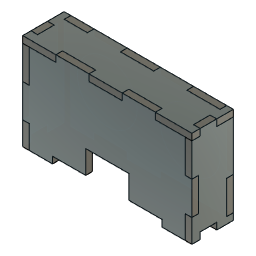
HR-SR04 LASER CUT PART v9 (Autodesk Fusion 360 design; units mm, degrees)
Autodesk Fusion 360 part; units mm, degrees
mesh "Mesh1" [no effect]
ref_plane "WorkPlane1" through (0, -8, 0) normal (0, 1, 0) x (0, 0, 1)
sketch "Sketch2" plane through (0, -8, 0) normal (0, 1, 0) x (1, 0, 0)
  line L0 (23.3967, -21.6051) -> (-23.6033, -21.6051)
  line L1 (-23.6033, -21.6051) -> (-23.6033, 3.3949)
  line L2 (-23.6033, 3.3949) -> (23.3967, 3.3949)
  line L3 (23.3967, 3.3949) -> (23.3967, -21.6051)
  line L4 (-23.6033, -9.1051) -> (-12.6033, -9.1051) construction
  line L5 (-12.6033, -9.1051) -> (-12.6033, 3.3949) construction
  line L6 (23.3967, -9.1051) -> (12.3967, -9.1051) construction
  line L7 (12.3967, -9.1051) -> (12.3967, 3.3949)
  circle A0 centre (12.3967, -9.1051) radius 9
  circle A1 centre (-12.6033, -9.1051) radius 9
  line L8 (23.3967, -21.6051) -> (23.3967, -23.6051)
  line L9 (23.3967, -23.6051) -> (13.3967, -23.6051)
  line L10 (13.3967, -23.6051) -> (13.3967, -21.6051)
  line L11 (13.3967, -21.6051) -> (23.3967, -21.6051)
  line L12 (3.3967, -23.6051) -> (-6.6033, -23.6051)
  line L13 (-6.6033, -23.6051) -> (-6.6033, -21.6051)
  line L14 (-6.6033, -21.6051) -> (3.3967, -21.6051)
  line L15 (3.3967, -21.6051) -> (3.3967, -23.6051)
  line L16 (-6.6033, -23.6051) -> (-16.6033, -23.6051) construction
  line L17 (-16.6033, -23.6051) -> (-16.6033, -21.6051)
  line L18 (-16.6033, -23.6051) -> (-23.6033, -23.6051)
  line L19 (-23.6033, -23.6051) -> (-23.6033, -21.6051)
  line L20 (23.3967, 3.3949) -> (25.3967, 3.3949)
  line L21 (25.3967, 3.3949) -> (25.3967, -6.6051)
  line L22 (25.3967, -6.6051) -> (23.3967, -6.6051)
  line L23 (23.3967, -6.6051) -> (23.3967, 3.3949)
  line L24 (23.3967, 3.3949) -> (23.3967, 5.3949)
  line L25 (23.3967, 5.3949) -> (13.3967, 5.3949)
  line L26 (13.3967, 5.3949) -> (13.3967, 3.3949)
  line L27 (13.3967, 3.3949) -> (23.3967, 3.3949)
  line L28 (3.3967, 5.3949) -> (-6.6033, 5.3949)
  line L29 (-6.6033, 5.3949) -> (-6.6033, 3.3949)
  line L30 (3.3967, 3.3949) -> (3.3967, 5.3949)
  line L31 (-23.6033, 5.3949) -> (-23.6033, 3.3949)
  line L32 (-16.6033, 5.3949) -> (-23.6033, 5.3949)
  line L33 (-16.6033, 5.3949) -> (-16.6033, 3.3949)
  line L34 (-6.6033, 3.3949) -> (3.3967, 3.3949)
  line L35 (-23.6033, -21.6051) -> (-25.6033, -21.6051)
  line L36 (-25.6033, -21.6051) -> (-25.6033, -11.6051)
  line L37 (-25.6033, -11.6051) -> (-23.6033, -11.6051)
  dimension "d2" = 47
  dimension "d3" = 25
  dimension "d4" = 11
  dimension "d5" = 11
  dimension "d6" = 18
  dimension "d7" = 18
  dimension "d14" = 2
  dimension "d15" = 10
  dimension "d16" = 2
  dimension "d20" = -20
  dimension "d21" = 0
  dimension "d25" = 10
  dimension "d26" = 2
  dimension "d30" = 2
  dimension "d31" = 10
  dimension "d37" = 2
  dimension "d38" = 10
  constraint horizontal L0
  constraint vertical L1
  constraint horizontal L2
  constraint vertical L3
  constraint midpoint L1 L4.start
  constraint perpendicular L1 L4
  constraint coincident L2 L5.end
  constraint perpendicular L2 L5
  constraint midpoint L3 L6.start
  constraint perpendicular L3 L6
  constraint coincident L2 L7.end
  constraint perpendicular L2 L7
  constraint coincident L6.end L7.start
  constraint coincident L4.end L5.start
  constraint perpendicular L0 L8
  constraint perpendicular L8 L9
  constraint perpendicular L0 L10
  constraint perpendicular L13 L16
  constraint perpendicular L0 L17
  constraint perpendicular L1 L18
  constraint perpendicular L0 L19
  constraint perpendicular L3 L20
  constraint perpendicular L20 L21
  constraint coincident L3 L22.end
  constraint perpendicular L3 L22
  constraint symmetric L0.start L4 L2.end
  constraint symmetric L0.end L4 L1.end
  constraint symmetric L4 L8.end L24.end
  constraint symmetric L4 L9.end L25.end
  constraint symmetric L4 L10.end L26.end
  constraint symmetric L4 L12.start L28.start
  constraint symmetric L4 L12.end L28.end
  constraint symmetric L4 L13.end L29.end
  constraint symmetric L4 L14.end L30.start
  constraint symmetric L4 L16.end L32.start
  constraint symmetric L4 L17.end L33.end
  constraint symmetric L4 L18.end L31.start
  constraint perpendicular L19 L35
  constraint perpendicular L35 L36
  constraint coincident L1 L37.end
  constraint perpendicular L1 L37
  measures "d2" distance of L0.start L0.end
  measures "d3" distance of L0.end L1.end
  measures "d4" distance of L4.start L4.end
  measures "d5" distance of L6.start L6.end
  measures "d6" diameter of A0
  measures "d7" diameter of A1
  measures "d14" distance of L0.start L8.end
  measures "d15" distance of L8.end L9.end
  measures "d16" distance of L9.end L10.end
  measures "d25" distance of L12.end L16.end
  measures "d26" distance of L16.end L17.end
  measures "d30" distance of L2.end L20.end
  measures "d31" distance of L20.end L21.end
  measures "d37" distance of L0.end L35.end
  measures "d38" distance of L35.end L36.end
extrude "Extrude1" add sketch "Sketch2" along normal blind 2 contours L0 L1 L2 L3 L11 L14 L23 L27 L34 makes body 1
extrude "Extrude2" add sketch "Sketch2" along normal blind 2 contours L0 L8 L9 L10 L11 | L0 L12 L13 L14 L15 bodies 1
extrude "Extrude3" add sketch "Sketch2" along normal blind 2 contours L0 L17 L18 L19 bodies 1
extrude "Extrude4" add sketch "Sketch2" along normal blind 2 contours L3 L20 L21 L22 L23 bodies 1
extrude "Extrude5" add sketch "Sketch2" along normal blind 2 contours L2 L24 L25 L26 L27 | L2 L28 L29 L30 L34 | L2 L31 L32 L33 bodies 1
extrude "Extrude6" add sketch "Sketch2" along normal blind 2 contours L1 L35 L36 L37 bodies 1
sketch "Sketch3" plane through (0, 0, 23.6051) normal (0, 0, 1) x (-1, 0, 0)
  line L0 (6.6033, 8) -> (-3.3967, 8)
  line L1 (-3.3967, 8) -> (-3.3967, 6)
  line L2 (-3.3967, 6) -> (6.6033, 6)
  line L3 (6.6033, 6) -> (6.6033, 8)
  line L4 (25.6033, 6) -> (-25.3967, 6)
  line L5 (-25.3967, 6) -> (-25.3967, 18.5)
  line L6 (-25.3967, 18.5) -> (25.6033, 18.5)
  line L7 (25.6033, 18.5) -> (25.6033, 6)
  line L8 (23.6033, 6) -> (16.6033, 6)
  line L9 (16.6033, 6) -> (16.6033, 8)
  line L10 (16.6033, 8) -> (23.6033, 8)
  line L11 (23.6033, 8) -> (23.6033, 6)
  line L12 (6.6033, 6) -> (-3.3967, 6)
  line L13 (-3.3967, 6) -> (-3.3967, 8)
  line L14 (-3.3967, 8) -> (6.6033, 8)
  line L15 (6.6033, 8) -> (6.6033, 6)
  line L16 (-13.3967, 6) -> (-23.3967, 6)
  line L17 (-23.3967, 6) -> (-23.3967, 8)
  line L18 (-23.3967, 8) -> (-13.3967, 8)
  line L19 (-13.3967, 8) -> (-13.3967, 6)
  line L20 (-25.3967, 6) -> (-25.3967, 11)
  line L21 (-25.3967, 11) -> (-23.3967, 11)
  line L22 (-23.3967, 11) -> (-23.3967, 16)
  line L23 (-23.3967, 16) -> (-25.3967, 16)
  line L24 (25.6033, 6) -> (25.6033, 11)
  line L25 (25.6033, 11) -> (23.6033, 11)
  line L26 (23.6033, 11) -> (23.6033, 16)
  line L27 (23.6033, 16) -> (25.6033, 16)
  line L28 (25.6033, 18.5) -> (15.6033, 18.5)
  line L29 (15.6033, 18.5) -> (15.6033, 16.5)
  line L30 (15.6033, 16.5) -> (5.6033, 16.5)
  line L31 (5.6033, 16.5) -> (5.6033, 18.5)
  line L32 (5.6033, 18.5) -> (-4.3967, 18.5)
  line L33 (-4.3967, 18.5) -> (-4.3967, 16.5)
  line L34 (-4.3967, 16.5) -> (-14.3967, 16.5)
  line L35 (-14.3967, 16.5) -> (-14.3967, 18.5)
  point P0 (25.6033, 6)
  point P1 (-25.3967, 6)
  point P2 (23.6033, 6)
  point P3 (16.6033, 8)
  point P4 (-13.3967, 6)
  point P5 (-23.3967, 8)
  dimension "d42" = 12.5
  dimension "d45" = 5
  dimension "d46" = 2
  dimension "d47" = 5
  dimension "d62" = 5
  dimension "d63" = 2
  dimension "d64" = 5
  dimension "d80" = 10
  dimension "d81" = 2
  dimension "d82" = 10
  dimension "d83" = 10
  dimension "d84" = 2
  dimension "d85" = 10
  constraint horizontal L4
  constraint vertical L5
  constraint horizontal L6
  constraint vertical L7
  constraint coincident P0 L4.start
  constraint coincident P1 L4.end
  constraint horizontal L8
  constraint vertical L9
  constraint horizontal L10
  constraint vertical L11
  constraint coincident P2 L8.start
  constraint coincident P3 L9.end
  constraint horizontal L12
  constraint vertical L13
  constraint horizontal L14
  constraint vertical L15
  constraint coincident L2.end L3.start
  constraint coincident L0.end L1.start
  constraint horizontal L16
  constraint vertical L17
  constraint horizontal L18
  constraint vertical L19
  constraint coincident P4 L16.start
  constraint coincident P5 L17.end
  constraint perpendicular L4 L20
  constraint perpendicular L20 L21
  constraint perpendicular L6 L22
  constraint coincident L5 L23.end
  constraint perpendicular L5 L23
  constraint perpendicular L4 L24
  constraint perpendicular L7 L25
  constraint perpendicular L25 L26
  constraint coincident L7 L27.end
  constraint perpendicular L7 L27
  constraint perpendicular L7 L28
  constraint perpendicular L6 L29
  constraint perpendicular L29 L30
  constraint coincident L6 L31.end
  constraint perpendicular L6 L31
  constraint perpendicular L31 L32
  constraint perpendicular L6 L33
  constraint perpendicular L33 L34
  constraint coincident L6 L35.end
  constraint perpendicular L6 L35
  measures "d42" distance of P1 L5.end
  measures "d45" distance of P1 L20.end
  measures "d46" distance of L20.end L21.end
  measures "d47" distance of L21.end L22.end
  measures "d62" distance of P0 L24.end
  measures "d63" distance of L24.end L25.end
  measures "d64" distance of L25.end L26.end
  measures "d80" distance of L6.end L28.end
  measures "d81" distance of L28.end L29.end
  measures "d82" distance of L29.end L30.end
  measures "d83" distance of L31.end L32.end
  measures "d84" distance of L32.end L33.end
  measures "d85" distance of L33.end L34.end
extrude "Extrude8" add sketch "Sketch3" against normal blind 2 separate body contours L0 L1 L3 L4 L5 L6 L7 L9 L10 L11 L13 L14 L15 L17 L18 L19 L20 L21 L22 L23 L24 L25 L26 L27 L28 L29 L30 L31 L32 L33 L34 L35 | L7 L25 L26 L27 | L6 L29 L30 L31 | L6 L33 L34 L35 makes body 2
sketch "Sketch4" plane through (23.3967, 0, 0) normal (1, 0, 0) x (0, 1, 0)
  line L0 (-8, 6.6051) -> (-6, 6.6051)
  line L1 (-6, 6.6051) -> (-6, 23.6051)
  line L2 (-6, 23.6051) -> (-8, 23.6051)
  line L3 (-8, 23.6051) -> (-8, 6.6051)
  line L4 (-18.5, 23.6051) -> (-6, 23.6051)
  line L5 (-6, 23.6051) -> (-6, -5.3949)
  line L6 (-6, -5.3949) -> (-18.5, -5.3949)
  line L7 (-18.5, -5.3949) -> (-18.5, 23.6051)
  line L8 (-18.5, 23.6051) -> (-16, 23.6051)
  line L9 (-16, 23.6051) -> (-16, 21.6051)
  line L10 (-16, 21.6051) -> (-18.5, 21.6051)
  line L11 (-18.5, 21.6051) -> (-18.5, 23.6051)
  line L12 (-11, 23.6051) -> (-6, 23.6051)
  line L13 (-6, 23.6051) -> (-6, 21.6051)
  line L14 (-6, 21.6051) -> (-11, 21.6051)
  line L15 (-11, 21.6051) -> (-11, 23.6051)
  line L16 (-8, 6.6051) -> (-6, 6.6051)
  line L17 (-6, 6.6051) -> (-6, -3.3949)
  line L18 (-6, -3.3949) -> (-8, -3.3949)
  line L19 (-8, -3.3949) -> (-8, 6.6051)
  line L20 (-18.5, 21.6051) -> (-18.5, 11.6051)
  line L21 (-18.5, 11.6051) -> (-16.5, 11.6051)
  line L22 (-16.5, 11.6051) -> (-16.5, 1.6051)
  line L23 (-16.5, 1.6051) -> (-18.5, 1.6051)
  line L24 (-6, -5.3949) -> (-11, -5.3949)
  line L25 (-11, -5.3949) -> (-11, -3.3949)
  line L26 (-11, -3.3949) -> (-16, -3.3949)
  line L27 (-16, -3.3949) -> (-16, -5.3949)
  point P0 (-18.5, 23.6051)
  point P1 (-6, 23.6051)
  point P2 (-6, -5.3949)
  point P3 (-16, 21.6051)
  point P4 (-11, 23.6051)
  point P5 (-6, 21.6051)
  point P6 (-6, -3.3949)
  dimension "d52" = 10
  dimension "d53" = 2
  dimension "d54" = 10
  dimension "d55" = 2
  dimension "d58" = 5
  dimension "d59" = 2
  dimension "d77" = 5
  constraint horizontal L4
  constraint vertical L5
  constraint horizontal L6
  constraint vertical L7
  constraint coincident P0 L4.start
  constraint coincident P1 L1.end
  constraint coincident P2 L5.end
  constraint horizontal L8
  constraint vertical L9
  constraint horizontal L10
  constraint vertical L11
  constraint coincident P3 L9.end
  constraint horizontal L12
  constraint vertical L13
  constraint horizontal L14
  constraint vertical L15
  constraint coincident P4 L12.start
  constraint coincident P5 L13.end
  constraint horizontal L16
  constraint vertical L17
  constraint horizontal L18
  constraint vertical L19
  constraint coincident L0.start L3.end
  constraint coincident P6 L17.end
  constraint perpendicular L6 L20
  constraint perpendicular L7 L21
  constraint perpendicular L21 L22
  constraint perpendicular L7 L23
  constraint perpendicular L5 L24
  constraint perpendicular L24 L25
  constraint perpendicular L25 L26
  constraint coincident L6 L27.end
  constraint perpendicular L6 L27
  measures "d52" distance of L10.end L20.end
  measures "d53" distance of L20.end L21.end
  measures "d54" distance of L21.end L22.end
  measures "d55" distance of L22.end L23.end
  measures "d58" distance of P2 L24.end
  measures "d59" distance of L24.end L25.end
  measures "d77" distance of L25.end L26.end
extrude "Extrude12" cut sketch "Sketch3" against normal blind 2 contours L7 L25 L26 L27 bodies 2
ref_plane "WorkPlane2" through (-0.1033, -17.25, 22.6051) normal (1, 0, 0) x (0, -1, 0)
sketch "Sketch5" plane through (-23.6033, 0, 0) normal (-1, 0, 0) x (0, -1, 0)
  line L0 (16, 23.6051) -> (11, 23.6051)
  line L1 (11, 23.6051) -> (11, 21.6051)
  line L2 (11, 21.6051) -> (16, 21.6051)
  line L3 (16, 21.6051) -> (16, 23.6051)
  line L4 (6, 23.6051) -> (18.5, 23.6051)
  line L5 (18.5, 23.6051) -> (18.5, -5.3949)
  line L6 (18.5, -5.3949) -> (6, -5.3949)
  line L7 (6, -5.3949) -> (6, 23.6051)
  line L8 (6, 11.6051) -> (8, 11.6051)
  line L9 (8, 11.6051) -> (8, 21.6051)
  line L10 (8, 21.6051) -> (6, 21.6051)
  line L11 (6, 21.6051) -> (6, 11.6051)
  line L12 (11, 21.6051) -> (6, 21.6051)
  line L13 (6, 21.6051) -> (6, 23.6051)
  line L14 (6, 23.6051) -> (11, 23.6051)
  line L15 (11, 23.6051) -> (11, 21.6051)
  line L16 (16, 21.6051) -> (18.5, 21.6051)
  line L17 (18.5, 21.6051) -> (18.5, 23.6051)
  line L18 (18.5, 23.6051) -> (16, 23.6051)
  line L19 (16, 23.6051) -> (16, 21.6051)
  line L20 (6, -5.3949) -> (11, -5.3949)
  line L21 (11, -5.3949) -> (11, -3.3949)
  line L22 (11, -3.3949) -> (16, -3.3949)
  line L23 (16, -3.3949) -> (16, -5.3949)
  line L24 (18.5, 21.6051) -> (18.5, 11.6051)
  line L25 (18.5, 11.6051) -> (16.5, 11.6051)
  line L26 (16.5, 11.6051) -> (16.5, 1.6051)
  line L27 (16.5, 1.6051) -> (18.5, 1.6051)
  point P0 (6, -5.3949)
  point P1 (18.5, 23.6051)
  point P2 (8, 11.6051)
  dimension "d69" = 5
  dimension "d70" = 2
  dimension "d71" = 5
  dimension "d72" = 10
  dimension "d73" = 2
  dimension "d74" = 10
  constraint horizontal L4
  constraint vertical L5
  constraint horizontal L6
  constraint vertical L7
  constraint coincident P0 L6.end
  constraint coincident P1 L4.end
  constraint horizontal L8
  constraint vertical L9
  constraint horizontal L10
  constraint vertical L11
  constraint coincident L7 L8.start
  constraint horizontal L12
  constraint vertical L13
  constraint horizontal L14
  constraint vertical L15
  constraint coincident L1.end L2.start
  constraint horizontal L16
  constraint vertical L17
  constraint horizontal L18
  constraint vertical L19
  constraint coincident L2.end L3.start
  constraint coincident L4.start L7.end
  constraint coincident P2 L8.end
  constraint coincident L9.end L12
  constraint perpendicular L7 L20
  constraint perpendicular L6 L21
  constraint perpendicular L21 L22
  constraint coincident L6 L23.end
  constraint perpendicular L6 L23
  constraint perpendicular L16 L24
  constraint perpendicular L24 L25
  constraint perpendicular L25 L26
  constraint coincident L5 L27.end
  constraint perpendicular L5 L27
  measures "d69" distance of P0 L20.end
  measures "d70" distance of L20.end L21.end
  measures "d71" distance of L21.end L22.end
  measures "d72" distance of L16.end L24.end
  measures "d73" distance of L24.end L25.end
  measures "d74" distance of L25.end L26.end
extrude "Extrude13" add sketch "Sketch5" along normal blind 2 separate body contours L0 L1 L2 L3 L4 L15 L19 | L2 L5 L6 L7 L8 L9 L12 L16 L20 L21 L22 L23 L24 L25 L26 L27 makes body 3
extrude "Extrude14" add sketch "Sketch4" along normal blind 2 separate body contours L0 L1 L3 L5 L14 L16 | L3 L4 L5 L6 L7 L9 L10 L14 L15 L18 L19 L20 L21 L22 L23 L24 L25 L26 L27 makes body 4
extrude "Extrude15" cut sketch "Sketch3" against normal blind 2 contours L6 L29 L30 L31 | L6 L33 L34 L35 bodies 2
sketch "Sketch7" plane through (0, -16.5, 0) normal (0, -1, 0) x (1, 0, 0)
  line L0 (-23.6033, 1.6051) -> (-23.6033, 11.6051)
  line L1 (-23.6033, 11.6051) -> (-25.6033, 11.6051)
  line L2 (-25.6033, 11.6051) -> (-25.6033, 1.6051)
  line L3 (-25.6033, 1.6051) -> (-23.6033, 1.6051)
  line L4 (-25.6033, 23.6051) -> (25.3967, 23.6051)
  line L5 (25.3967, 23.6051) -> (25.3967, -5.3949)
  line L6 (-25.6033, -5.3949) -> (-25.6033, 23.6051)
  line L7 (-25.6033, 11.6051) -> (-23.6033, 11.6051)
  line L8 (-23.6033, 11.6051) -> (-23.6033, 21.6051)
  line L9 (-23.6033, 21.6051) -> (-25.6033, 21.6051)
  line L10 (-25.6033, 21.6051) -> (-25.6033, 11.6051)
  line L11 (-25.6033, 21.6051) -> (-15.6033, 21.6051)
  line L12 (-15.6033, 21.6051) -> (-15.6033, 23.6051)
  line L13 (-15.6033, 23.6051) -> (-25.6033, 23.6051)
  line L14 (-25.6033, 23.6051) -> (-25.6033, 21.6051)
  line L15 (-5.6033, 23.6051) -> (4.3967, 23.6051)
  line L16 (4.3967, 23.6051) -> (4.3967, 21.6051)
  line L17 (4.3967, 21.6051) -> (-5.6033, 21.6051)
  line L18 (-5.6033, 21.6051) -> (-5.6033, 23.6051)
  line L19 (14.3967, 23.6051) -> (25.3967, 23.6051)
  line L20 (25.3967, 23.6051) -> (25.3967, 21.6051)
  line L21 (25.3967, 21.6051) -> (14.3967, 21.6051)
  line L22 (14.3967, 21.6051) -> (14.3967, 23.6051)
  line L23 (23.3967, 21.6051) -> (25.3967, 21.6051)
  line L24 (25.3967, 21.6051) -> (25.3967, 11.6051)
  line L25 (25.3967, 11.6051) -> (23.3967, 11.6051)
  line L26 (23.3967, 11.6051) -> (23.3967, 21.6051)
  line L27 (23.3967, 1.6051) -> (25.3967, 1.6051)
  line L28 (25.3967, 1.6051) -> (25.3967, -5.3949)
  line L29 (25.3967, -5.3949) -> (23.3967, -5.3949)
  line L30 (23.3967, -5.3949) -> (23.3967, 1.6051)
  line L31 (-25.6033, -5.3949) -> (-23.6033, -5.3949)
  line L32 (-23.6033, -5.3949) -> (-23.6033, 1.6051)
  line L33 (-23.6033, 1.6051) -> (-25.6033, 1.6051)
  line L34 (-25.6033, 1.6051) -> (-25.6033, -5.3949)
  line L35 (6.3967, 3.6051) -> (-6.6033, 3.6051)
  line L36 (-6.6033, 3.6051) -> (-6.6033, -5.3949)
  line L37 (-0.1033, 23.6051) -> (-0.1033, 3.6051) construction
  line L38 (6.3967, 3.6051) -> (6.3967, -5.3949)
  line L39 (-25.6033, -5.3949) -> (25.3967, -5.3949)
  line L40 (-6.6033, -5.3949) -> (-16.6033, -5.3949)
  line L41 (-16.6033, -5.3949) -> (-16.6033, -3.3949)
  line L42 (-16.6033, -3.3949) -> (-6.6033, -3.3949)
  line L43 (-6.6033, -3.3949) -> (-6.6033, -5.3949)
  line L44 (6.3967, -5.3949) -> (16.3967, -5.3949)
  line L45 (16.3967, -5.3949) -> (16.3967, -3.3949)
  line L46 (16.3967, -3.3949) -> (6.3967, -3.3949)
  line L47 (6.3967, -3.3949) -> (6.3967, -5.3949)
  point P0 (-25.6033, 23.6051)
  point P1 (25.3967, -5.3949)
  point P2 (-23.6033, 21.6051)
  point P3 (-15.6033, 23.6051)
  point P4 (-5.6033, 21.6051)
  point P5 (4.3967, 23.6051)
  point P6 (14.3967, 21.6051)
  point P7 (23.3967, 21.6051)
  point P8 (25.3967, 11.6051)
  point P9 (23.3967, 1.6051)
  dimension "d96" = 20
  dimension "d97" = 13
  dimension "d98" = 10
  dimension "d99" = 2
  dimension "d100" = 10
  dimension "d101" = 2
  constraint horizontal L4
  constraint vertical L5
  constraint vertical L6
  constraint coincident P0 L4.start
  constraint coincident P1 L5.end
  constraint horizontal L7
  constraint vertical L8
  constraint horizontal L9
  constraint vertical L10
  constraint coincident L1.end L2.start
  constraint coincident P2 L8.end
  constraint horizontal L11
  constraint vertical L12
  constraint horizontal L13
  constraint vertical L14
  constraint coincident P3 L12.end
  constraint horizontal L15
  constraint vertical L16
  constraint horizontal L17
  constraint vertical L18
  constraint coincident P4 L17.end
  constraint coincident P5 L15.end
  constraint horizontal L19
  constraint vertical L20
  constraint horizontal L21
  constraint vertical L22
  constraint coincident P6 L21.end
  constraint coincident L4.end L5.start
  constraint horizontal L23
  constraint vertical L24
  constraint horizontal L25
  constraint vertical L26
  constraint coincident P7 L23.start
  constraint coincident P8 L24.end
  constraint horizontal L27
  constraint vertical L28
  constraint horizontal L29
  constraint vertical L30
  constraint coincident P9 L27.start
  constraint horizontal L31
  constraint vertical L32
  constraint horizontal L33
  constraint vertical L34
  constraint coincident L0.start L3.end
  constraint horizontal L35
  constraint vertical L36
  constraint midpoint L4 L37.start
  constraint midpoint L35 L37.end
  constraint perpendicular L17 L37
  constraint perpendicular L35 L38
  constraint perpendicular L28 L39
  constraint horizontal L40
  constraint vertical L41
  constraint horizontal L42
  constraint vertical L43
  constraint collinear L39 L40
  constraint horizontal L44
  constraint vertical L45
  constraint horizontal L46
  constraint vertical L47
  constraint collinear L39 L44
  measures "d96" distance of L37.start L37.end
  measures "d97" distance of L35.start L35.end
  measures "d98" distance of L36.end L40.end
  measures "d99" distance of L36.end L42.end
  measures "d100" distance of L38.end L44.end
  measures "d101" distance of L38.end L46.end
extrude "Extrude18" add sketch "Sketch7" along normal blind 2 separate body contours L0 L1 L2 L3 L6 L7 L33 | L0 L4 L5 L8 L11 L12 L16 L17 L18 L21 L22 L25 L26 L27 L30 L32 L35 L36 L38 L39 L41 L42 L45 L46 makes body 5
sketch "FRONT_DXF" plane through (0, -6, 0) normal (0, 1, 0) x (-1, 0, 0)
  circle A0 centre (12.6033, 9.1051) radius 9
  circle A1 centre (-12.3967, 9.1051) radius 9
  line L0 (16.6033, 21.6051) -> (6.6033, 21.6051)
  line L1 (6.6033, 21.6051) -> (6.6033, 23.6051)
  line L2 (6.6033, 23.6051) -> (-3.3967, 23.6051)
  line L3 (-3.3967, 23.6051) -> (-3.3967, 21.6051)
  line L4 (-3.3967, 21.6051) -> (-13.3967, 21.6051)
  line L5 (-13.3967, 21.6051) -> (-13.3967, 23.6051)
  line L6 (-13.3967, 23.6051) -> (-23.3967, 23.6051)
  line L7 (-23.3967, 23.6051) -> (-23.3967, 6.6051)
  line L8 (-23.3967, 6.6051) -> (-25.3967, 6.6051)
  line L9 (-25.3967, 6.6051) -> (-25.3967, -3.3949)
  line L10 (-25.3967, -3.3949) -> (-23.3967, -3.3949)
  line L11 (-23.3967, -3.3949) -> (-23.3967, -5.3949)
  line L12 (-23.3967, -5.3949) -> (-13.3967, -5.3949)
  line L13 (-13.3967, -5.3949) -> (-13.3967, -3.3949)
  line L14 (-13.3967, -3.3949) -> (-3.3967, -3.3949)
  line L15 (-3.3967, -3.3949) -> (-3.3967, -5.3949)
  line L16 (-3.3967, -5.3949) -> (6.6033, -5.3949)
  line L17 (6.6033, -5.3949) -> (6.6033, -3.3949)
  line L18 (6.6033, -3.3949) -> (16.6033, -3.3949)
  line L19 (16.6033, -3.3949) -> (16.6033, -5.3949)
  line L20 (16.6033, -5.3949) -> (23.6033, -5.3949)
  line L21 (23.6033, -5.3949) -> (23.6033, 11.6051)
  line L22 (23.6033, 11.6051) -> (25.6033, 11.6051)
  line L23 (25.6033, 11.6051) -> (25.6033, 21.6051)
  line L24 (25.6033, 21.6051) -> (23.6033, 21.6051)
  line L25 (23.6033, 21.6051) -> (23.6033, 23.6051)
  line L26 (23.6033, 23.6051) -> (16.6033, 23.6051)
  line L27 (16.6033, 23.6051) -> (16.6033, 21.6051)
sketch "LEFT_DXF" plane through (25.3967, 0, 0) normal (1, 0, 0) x (0, 1, 0)
  line L0 (-6, -3.3949) -> (-8, -3.3949)
  line L1 (-8, -3.3949) -> (-8, 6.6051)
  line L2 (-8, 6.6051) -> (-6, 6.6051)
  line L3 (-6, 6.6051) -> (-6, 21.6051)
  line L4 (-6, 21.6051) -> (-11, 21.6051)
  line L5 (-11, 21.6051) -> (-11, 23.6051)
  line L6 (-11, 23.6051) -> (-16, 23.6051)
  line L7 (-16, 23.6051) -> (-16, 21.6051)
  line L8 (-16, 21.6051) -> (-18.5, 21.6051)
  line L9 (-18.5, 21.6051) -> (-18.5, 11.6051)
  line L10 (-18.5, 11.6051) -> (-16.5, 11.6051)
  line L11 (-16.5, 11.6051) -> (-16.5, 1.6051)
  line L12 (-16.5, 1.6051) -> (-18.5, 1.6051)
  line L13 (-18.5, 1.6051) -> (-18.5, -5.3949)
  line L14 (-18.5, -5.3949) -> (-16, -5.3949)
  line L15 (-16, -5.3949) -> (-16, -3.3949)
  line L16 (-16, -3.3949) -> (-11, -3.3949)
  line L17 (-11, -3.3949) -> (-11, -5.3949)
  line L18 (-11, -5.3949) -> (-6, -5.3949)
  line L19 (-6, -5.3949) -> (-6, -3.3949)
sketch "RIGHT_DXF" plane through (-25.6033, 0, 0) normal (-1, 0, 0) x (0, -1, 0)
  line L0 (11, 23.6051) -> (11, 21.6051)
  line L1 (11, 21.6051) -> (8, 21.6051)
  line L2 (8, 21.6051) -> (8, 11.6051)
  line L3 (8, 11.6051) -> (6, 11.6051)
  line L4 (6, 11.6051) -> (6, -5.3949)
  line L5 (6, -5.3949) -> (11, -5.3949)
  line L6 (11, -5.3949) -> (11, -3.3949)
  line L7 (11, -3.3949) -> (16, -3.3949)
  line L8 (16, -3.3949) -> (16, -5.3949)
  line L9 (16, -5.3949) -> (18.5, -5.3949)
  line L10 (18.5, -5.3949) -> (18.5, 1.6051)
  line L11 (18.5, 1.6051) -> (16.5, 1.6051)
  line L12 (16.5, 1.6051) -> (16.5, 11.6051)
  line L13 (16.5, 11.6051) -> (18.5, 11.6051)
  line L14 (18.5, 11.6051) -> (18.5, 21.6051)
  line L15 (18.5, 21.6051) -> (16, 21.6051)
  line L16 (16, 21.6051) -> (16, 23.6051)
  line L17 (16, 23.6051) -> (11, 23.6051)
sketch "TOP_DXF" plane through (0, 0, 23.6051) normal (0, 0, 1) x (-1, 0, 0)
  line L0 (5.6033, 16.5) -> (5.6033, 18.5)
  line L1 (5.6033, 18.5) -> (-4.3967, 18.5)
  line L2 (-4.3967, 18.5) -> (-4.3967, 16.5)
  line L3 (-4.3967, 16.5) -> (-14.3967, 16.5)
  line L4 (-14.3967, 16.5) -> (-14.3967, 18.5)
  line L5 (-14.3967, 18.5) -> (-25.3967, 18.5)
  line L6 (-25.3967, 18.5) -> (-25.3967, 16)
  line L7 (-25.3967, 16) -> (-23.3967, 16)
  line L8 (-23.3967, 16) -> (-23.3967, 11)
  line L9 (-23.3967, 11) -> (-25.3967, 11)
  line L10 (-25.3967, 11) -> (-25.3967, 6)
  line L11 (-25.3967, 6) -> (-23.3967, 6)
  line L12 (-23.3967, 6) -> (-23.3967, 8)
  line L13 (-23.3967, 8) -> (-13.3967, 8)
  line L14 (-13.3967, 8) -> (-13.3967, 6)
  line L15 (-13.3967, 6) -> (-3.3967, 6)
  line L16 (-3.3967, 6) -> (-3.3967, 8)
  line L17 (-3.3967, 8) -> (6.6033, 8)
  line L18 (6.6033, 8) -> (6.6033, 6)
  line L19 (6.6033, 6) -> (16.6033, 6)
  line L20 (16.6033, 6) -> (16.6033, 8)
  line L21 (16.6033, 8) -> (23.6033, 8)
  line L22 (23.6033, 8) -> (23.6033, 6)
  line L23 (23.6033, 6) -> (25.6033, 6)
  line L24 (25.6033, 6) -> (25.6033, 11)
  line L25 (25.6033, 11) -> (23.6033, 11)
  line L26 (23.6033, 11) -> (23.6033, 16)
  line L27 (23.6033, 16) -> (25.6033, 16)
  line L28 (25.6033, 16) -> (25.6033, 18.5)
  line L29 (25.6033, 18.5) -> (15.6033, 18.5)
  line L30 (15.6033, 18.5) -> (15.6033, 16.5)
  line L31 (15.6033, 16.5) -> (5.6033, 16.5)
sketch "BACK_DXF" plane through (0, -18.5, 0) normal (0, -1, 0) x (1, 0, 0)
  line L0 (16.3967, -5.3949) -> (23.3967, -5.3949)
  line L1 (23.3967, -5.3949) -> (23.3967, 1.6051)
  line L2 (23.3967, 1.6051) -> (25.3967, 1.6051)
  line L3 (25.3967, 1.6051) -> (25.3967, 11.6051)
  line L4 (25.3967, 11.6051) -> (23.3967, 11.6051)
  line L5 (23.3967, 11.6051) -> (23.3967, 21.6051)
  line L6 (23.3967, 21.6051) -> (14.3967, 21.6051)
  line L7 (14.3967, 21.6051) -> (14.3967, 23.6051)
  line L8 (14.3967, 23.6051) -> (4.3967, 23.6051)
  line L9 (4.3967, 23.6051) -> (4.3967, 21.6051)
  line L10 (4.3967, 21.6051) -> (-5.6033, 21.6051)
  line L11 (-5.6033, 21.6051) -> (-5.6033, 23.6051)
  line L12 (-5.6033, 23.6051) -> (-15.6033, 23.6051)
  line L13 (-15.6033, 23.6051) -> (-15.6033, 21.6051)
  line L14 (-15.6033, 21.6051) -> (-23.6033, 21.6051)
  line L15 (-23.6033, 21.6051) -> (-23.6033, 11.6051)
  line L16 (-23.6033, 11.6051) -> (-25.6033, 11.6051)
  line L17 (-25.6033, 11.6051) -> (-25.6033, 1.6051)
  line L18 (-25.6033, 1.6051) -> (-23.6033, 1.6051)
  line L19 (-23.6033, 1.6051) -> (-23.6033, -5.3949)
  line L20 (-23.6033, -5.3949) -> (-16.6033, -5.3949)
  line L21 (-16.6033, -5.3949) -> (-16.6033, -3.3949)
  line L22 (-16.6033, -3.3949) -> (-6.6033, -3.3949)
  line L23 (-6.6033, -3.3949) -> (-6.6033, 3.6051)
  line L24 (-6.6033, 3.6051) -> (6.3967, 3.6051)
  line L25 (6.3967, 3.6051) -> (6.3967, -3.3949)
  line L26 (6.3967, -3.3949) -> (16.3967, -3.3949)
  line L27 (16.3967, -3.3949) -> (16.3967, -5.3949)
equation "d3 = usw"
equation "d8 = thick"
equation "slotl = 10 mm"
equation "slotw = 2 mm"
equation "usl = 47 mm"
equation "d14 = slotw"
equation "d15 = slotl"
equation "d16 = slotw"
equation "usls = usl / slotl / 2 - 0.35"
equation "d18 = usls"
equation "d20 = -slotl * 2"
equation "d22 = thick"
equation "thick = 2 mm"
equation "d26 = slotw"
equation "d27 = thick"
equation "usw = 25 mm"
equation "d30 = slotw"
equation "d31 = slotl"
equation "usws = usw / slotl / 2 - 0.1"
equation "d33 = thick"
equation "d35 = thick"
equation "d37 = slotw"
equation "d38 = slotl"
equation "d39 = thick"
equation "width = 12.5 mm"
equation "d42 = width"
equation "d45 = slotl / 2"
equation "d46 = slotw"
equation "d47 = slotl / 2"
equation "d48 = -thick"
equation "d52 = slotl"
equation "d53 = slotw"
equation "d54 = slotl"
equation "d55 = slotw"
equation "d58 = slotl / 2"
equation "d59 = slotw"
equation "d62 = slotl / 2"
equation "d63 = slotw"
equation "d64 = slotl / 2"
equation "d65 = -thick"
equation "d69 = slotl / 2"
equation "d70 = slotw"
equation "d71 = slotl / 2"
equation "d72 = slotl"
equation "d73 = slotw"
equation "d74 = slotl"
equation "d75 = thick"
equation "d77 = slotl / 2"
equation "d78 = thick"
equation "d80 = slotl"
equation "d81 = slotw"
equation "d82 = slotl"
equation "d83 = slotl"
equation "d84 = slotw"
equation "d85 = slotl"
equation "d86 = -thick"
equation "d98 = slotl"
equation "d99 = slotw"
equation "d100 = slotl"
equation "d101 = slotw"
equation "d104 = thick"
named bodies: "FRONT", "TOP", "RIGHT", "LEFT", "BACK"
